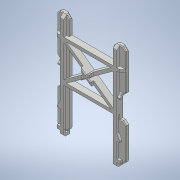
# Autodesk Inventor part: Крепление лидара
Saved by Autodesk Inventor 2020 (Build 240168000, 168)
## iProperties
Created: 2021-05-27
Part Number: Крепление лидара
Material: Типовые
Document SubType Name: Modeling
Designer: I_Love_U_Bogdan
Density: 1 g/cm^3
Appearance: По умолчанию
Author: I_Love_U_Bogdan
Autodesk Inventor part; units mm, degrees
ref_plane "YZ Plane" through (0, 0, 0) normal (1, 0, 0) x (0, 1, 0)
ref_plane "XZ Plane" through (0, 0, 0) normal (0, 1, 0) x (-1, 0, 0)
ref_plane "XY Plane" through (0, 0, 0) normal (0, 0, 1) x (1, 0, 0)
sketch "Эскиз1" plane through (0, 0, 0) normal (0, 0, 1) x (1, 0, 0)
  line L0 (-15, 85.8768) -> (-23, 85.8768)
  line L1 (-23, 85.8768) -> (-23, 17.8768)
  line L2 (-23, 17.8768) -> (-15, 17.8768)
  line L3 (-23.1, 75.8182) -> (-23.1, 81.8182) projected
  line L4 (-15, 85.8768) -> (-15, 17.8768)
  line L5 (-24.4209, 83.8768) -> (-19.4401, 83.8768) projected
  line L6 (-19.4401, 73.7596) -> (-24.4209, 73.7596) projected
  line L7 (-19.1, 75.8182) -> (-19.1, 81.8182) projected
  line L8 (-23, 57.8768) -> (-19, 57.8768)
  line L9 (-19, 57.8768) -> (-19, 42.8768)
  line L10 (-19, 42.8768) -> (-23, 42.8768)
  line L11 (-23, 42.8768) -> (-23, 57.8768)
  point P0 (0, 0)
  dimension "d0" = 0.1
  dimension "d1" = 68
  dimension "d2" = 8
  dimension "d3" = 2
  dimension "d4" = 10.1172
  dimension "d5" = 3.9
  dimension "d6" = 15
  dimension "d7" = 25
  constraints: 16 end point, 3 parallel, 2 horizontal, 2 perpendicular, 1 point on line
  measures "d0" distance between parallel lines of L3 L1
  measures "d1" distance of L0.end L1.end
  measures "d2" distance between parallel lines of L4 L1
  measures "d3" distance between parallel lines of L0 L5
  measures "d4" distance between parallel lines of L6 L5
  measures "d5" distance between parallel lines of L1 L7
  measures "d6" distance of L8.end L9.end
  measures "d7" distance between parallel lines of L2 L10
extrude "Выдавливание1" add sketch "Эскиз1" along normal blind 2 contours L4 L2 L1 L10 L9 L8 L0
sketch "Эскиз2" plane through (0, 0, 2) normal (0, 0, 1) x (1, 0, 0)
  line L0 (-19.4401, 73.7596) -> (-24.4209, 73.7596) projected
  line L1 (-23, 85.8768) -> (-23, 57.8768) projected
  line L2 (-23, 73.7596) -> (0, 73.7596)
  line L3 (0, 73.7596) -> (0, 71.7596)
  line L4 (0, 71.7596) -> (-23, 71.7596)
  line L5 (-23, 71.7596) -> (-23, 73.7596)
  line L6 (-15, 85.8768) -> (-23, 85.8768) projected
  line L7 (-15, 85.8768) -> (-16.5, 85.8768)
  line L8 (-16.5, 17.8768) -> (-15, 17.8768)
  line L9 (-19.1, 75.8182) -> (-19.1, 81.8182) projected
  line L10 (-25.5, 75.3182) -> (-26.5, 75.3182) projected
  line L11 (-23, 42.8768) -> (-23, 17.8768) projected
  line L12 (-23, 20.7596) -> (-19.1, 20.7596)
  line L13 (-25.5, 22.3182) -> (-26.5, 22.3182) projected
  line L14 (-26.5, 29.3182) -> (-25.5, 29.3182) projected
  line L15 (-23, 30.8768) -> (-19.1, 30.8768)
  line L16 (-16.5, 20.7596) -> (-21.1, 20.7596)
  line L17 (-21.1, 20.7596) -> (-21.1, 18.7596)
  line L18 (-21.1, 18.7596) -> (-16.5, 18.7596)
  line L19 (-23, 17.8768) -> (-15, 17.8768) projected
  line L20 (-16.5, 85.8768) -> (-19, 85.8768)
  line L21 (-19, 85.8768) -> (-19, 17.8768)
  line L22 (-19, 17.8768) -> (-16.5, 17.8768)
  line L23 (-16.5, 17.8768) -> (-16.5, 85.8768)
  line L24 (-21, 31.1768) -> (-21, 32.1768)
  line L25 (-21, 32.1768) -> (-19, 35.6409)
  line L26 (-16.5, 47.8768) -> (0, 47.8768)
  line L27 (0, 47.8768) -> (0, 45.8768)
  line L28 (0, 45.8768) -> (-16.5, 45.8768)
  line L29 (-16.5, 45.8768) -> (-16.5, 47.8768)
  line L30 (0, 71.7596) -> (0, 47.8768)
  line L31 (0, 59.8182) -> (-16.5, 47.8768) construction
  line L32 (-15.9137, 47.0667) -> (0.5863, 59.0081)
  arc A0 (0.5863, 59.0081) -> (0, 60.8182) centre (0, 59.8182) ccw
  arc A1 (-17.0863, 48.6869) -> (-15.9137, 47.0667) centre (-16.5, 47.8768) ccw
  line L33 (0, 59.8182) -> (-16.5, 71.7596) construction
  line L34 (0.5863, 60.6283) -> (-15.9137, 72.5697)
  arc A2 (0, 58.8182) -> (0.5863, 60.6283) centre (0, 59.8182) ccw
  arc A3 (-15.9137, 72.5697) -> (-17.0863, 70.9495) centre (-16.5, 71.7596) ccw
  line L35 (-17.0863, 70.9495) -> (-1.7056, 59.8182)
  line L36 (-1.7056, 59.8182) -> (-17.0863, 48.6869)
  line L37 (-21, 31.1768) -> (-19, 31.1768)
  line L38 (-19.1, 81.8182) -> (-19.1, 35.4676)
  line L39 (-19.1, 30.8768) -> (-19.1, 19.0812)
  point P0 (0, 0)
  point P1 (-8.25, 53.8475)
  point P2 (-8.25, 65.7889)
  point P3 (-16.5, 70.5252)
  point P4 (-16.5, 49.1112)
  point P5 (-14.7944, 71.7596)
  point P6 (-16.5, 73.7596)
  point P7 (-19, 20.7596)
  point P8 (-19, 18.7596)
  point P9 (-14.7944, 47.8768)
  point P10 (0, 58.5838)
  point P11 (0, 61.0526)
  point P12 (-19, 71.7596)
  point P13 (-19, 73.7596)
  dimension "d10" = 2
  dimension "d12" = 1.5586
  dimension "d13" = 1.5586
  dimension "d14" = 1.5586
  dimension "d15" = 2
  dimension "d16" = 0
  dimension "d18" = 2.5
  dimension "d22" = 30
  dimension "d23" = 1
  dimension "d24" = 2
  dimension "d25" = 2
  dimension "d26" = 2
  dimension "d27" = 28
  dimension "d30" = 0.3
  dimension "d56" = 0.1
  dimension "d57" = 0
  dimension "d59" = 2
  constraints: 66 end point, 16 point on line, 12 parallel, 9 perpendicular, 8 point on circle, 8 tangent, 5 horizontal, 4 centre point, 4 midpoint, 3 vertical
  measures "d10" distance of L2.end L3.end
  measures "d12" distance between parallel lines of L10 L0
  measures "d13" distance between parallel lines of L13 L12
  measures "d14" distance between parallel lines of L15 L14
  measures "d15" distance of L16.end L17.end
  measures "d16" distance between parallel lines of L12 L16
  measures "d18" distance between parallel lines of L23 L21
  measures "d22" angle of L25 L21
  measures "d23" distance of L24.start L24.end
  measures "d24" distance of L26.end L27.end
  measures "d25" diameter of A1
  measures "d26" diameter of A3
  measures "d27" distance between parallel lines of L19 L28
  measures "d30" distance between parallel lines of L15 L37
  measures "d56" distance between parallel lines of L21 L38
  measures "d57" horizontal distance of point (0, 0) L2.end
  measures "d59" distance between parallel lines of L21 L24
extrude "Выдавливание2" add sketch "Эскиз2" along normal blind 2 contours L2 L38 L4 L1 L0 | L2 L21 L4 L38 | L21 L6 L23 L2 | L2 L23 A3 L4 L21 | L2 L3 L4 L34 A3 L23 | L4 A3 L35 L23 L36 A1 L16 L21 | L25 L21 L37 L24 | A3 L34 L4 L23 | L23 L4 A3 | L4 L23 L35 A3 | L4 L34 L30 L32 L26 L23 L36 L35 | L21 L18 L17 L12 L16 | L16 L23 L18 L21 | L23 A1 L36 | L18 L23 L19 L21 | L26 L32 A1 L23 | L23 A1 L32 L26 L27 L28
sketch "Эскиз3" plane through (0, 0, 2) normal (0, 0, -1) x (-1, 0, 0)
  line L0 (16.5, 73.7596) -> (16.5, 85.8768) projected
  line L1 (16.5, 85.8768) -> (19, 85.8768) projected
  line L2 (19, 85.8768) -> (19, 73.7596) projected
  line L3 (19, 35.6409) -> (21, 32.1768) projected
  line L4 (21, 32.1768) -> (21, 31.1768) projected
  line L5 (21, 31.1768) -> (19, 31.1768) projected
  line L6 (19, 31.1768) -> (19, 20.7596) projected
  line L7 (19, 20.7596) -> (21.1, 20.7596) projected
  line L8 (21.1, 20.7596) -> (21.1, 18.7596) projected
  line L9 (21.1, 18.7596) -> (19, 18.7596) projected
  line L10 (19, 18.7596) -> (19, 17.8768) projected
  line L11 (19, 17.8768) -> (16.5, 17.8768) projected
  line L12 (16.5, 17.8768) -> (16.5, 45.8768) projected
  line L13 (16.5, 45.8768) -> (0, 45.8768) projected
  line L14 (0, 45.8768) -> (0, 47.8768) projected
  line L15 (0, 47.8768) -> (14.7944, 47.8768) projected
  line L16 (14.7944, 47.8768) -> (0, 58.5838) projected
  line L17 (0, 58.5838) -> (0, 61.0526) projected
  line L18 (0, 61.0526) -> (14.7944, 71.7596) projected
  line L19 (14.7944, 71.7596) -> (0, 71.7596) projected
  line L20 (0, 71.7596) -> (0, 73.7596) projected
  line L21 (0, 73.7596) -> (16.5, 73.7596) projected
  line L22 (1.7056, 59.8182) -> (16.5, 49.1112) projected
  line L23 (16.5, 49.1112) -> (16.5, 70.5252) projected
  line L24 (16.5, 70.5252) -> (1.7056, 59.8182) projected
  line L25 (15, 73.7596) -> (15, 85.8768) projected
  line L26 (15, 50.1967) -> (15, 69.4396) projected
  line L27 (15, 17.8768) -> (15, 45.8768) projected
  line L28 (15, 69.4396) -> (15, 73.7596) projected
  line L29 (15, 73.7596) -> (15, 45.8768)
  line L30 (15, 17.8768) -> (15, 85.8768) projected
  line L31 (19, 73.7596) -> (23, 73.7596) projected
  line L32 (23, 73.7596) -> (23, 71.7596) projected
  line L33 (23, 71.7596) -> (19, 71.7596) projected
  line L34 (19, 71.7596) -> (19, 35.6409) projected
  point P0 (0, 0)
  point P1 (15, 71.7596)
  point P2 (14.8, 47.8768)
  point P3 (14.8, 48.3873)
  point P4 (15, 50.1967)
  point P5 (14.8, 71.2491)
  constraints: 2 end point, 1 collinear
extrude "Выдавливание3" add sketch "Эскиз3" along normal blind 2 contours L0 L1 L2 L31 L32 L33 L34 L3 L4 L5 L6 L7 L8 L9 L10 L11 L12 L13 L29 L22 L23 L24 L28 L21 | L28 L24 L22 L29 L13 L14 L15 L16 L17 L18 L19 L20 L21 | L24 L23 L22 L26
chamfer "Фаска1" distance 2 angle 45 8 edges at (-23, 72.7596, 4) (-23, 85.8768, 1) (-17.75, 85.8768, 4) (-15, 85.8768, 1) (-15, 17.8768, 1) (-23, 17.8768, 1) (-23, 57.8768, 1) (-23, 42.8768, 1)
chamfer "Фаска2" distance 0.5 angle 45 17 edges at (-23, 78.8182, 2) (-23, 65.8182, 2) (-23, 30.3768, 2) (-22, 84.8768, 2) (-20, 85.8768, 2) (-15.75, 84.6268, 2) (-22, 84.8768, 0) (-16, 84.8768, 0) (-22, 18.8768, 0) (-22, 18.8768, 2) (-20, 17.8768, 2) (-15.75, 19.1268, 2) (-16, 18.8768, 0) (-20, 42.8768, 2) (-22, 41.8768, 2) (-20, 57.8768, 2) (-22, 58.8768, 2)
sketch "Эскиз7" plane through (-19, 17.8768, 4) normal (0, -1, 0) x (1, 0, 0)
  line L0 (2, -3.5) -> (1.2929, -4) projected
  line L1 (2, 0) -> (2, -3.5) projected
  line L2 (0, 0) -> (2, 0) projected
  line L3 (0, -2.5) -> (0, 0) projected
  line L4 (-2, -2.5) -> (0, -2.5) projected
  line L5 (-2, -3.5) -> (-2, -2.5) projected
  line L6 (-1.2929, -4) -> (-2, -3.5) projected
  line L7 (-1.2929, -4) -> (1.2929, -4) projected
  line L8 (0, 0) -> (2.5, 0) projected
  line L9 (4, -4) -> (1.2929, -4) projected
  line L10 (0, 0) -> (2.5231, 0)
  line L11 (2.5231, 0) -> (2.5231, -4)
  line L12 (2.5231, -4) -> (0, -4)
  line L13 (0, -4) -> (0, 0)
  point P0 (19, -4)
  point P1 (0, -4)
  constraints: 8 end point, 2 parallel, 1 horizontal, 1 perpendicular, 1 point on line
extrude "Выдавливание7" add sketch "Эскиз7" along normal mid plane 4 contours L1 L8 L10 L11 L9 L0 | L0 L7 L13 L3 L2 L1
chamfer "Фаска3" distance 1 angle 45 1 edges at (-17.7385, 15.8768, 4)
sketch "Эскиз4" plane through (-19, 20.7596, 2) normal (-1, 0, 0) x (0, 0, 1)
  line L0 (-2, 25.1172) -> (2, 25.1172) projected
  line L1 (-0.5, -2.8828) -> (2, -2.8828) projected
  line L2 (0, 25.1172) -> (0.6, 25.1172)
  line L3 (0.6, 25.1172) -> (0.6, -2.8828)
  line L4 (0.6, -2.8828) -> (0, -2.8828)
  line L5 (0, -2.8828) -> (0, 25.1172)
  line L6 (0, -2.3828) -> (-0.5, -2.8828) projected
  line L7 (-1.5, -2.8828) -> (-0.5, -2.8828) projected
  line L8 (-1.5, -3.2828) -> (-0.5, -3.2828)
  line L9 (0, -2.8828) -> (0, -3.2828)
  line L10 (0, -3.2828) -> (-0.5, -3.2828)
  line L11 (0.6, -2.8828) -> (0.6, -3.2828)
  line L12 (0.6, -3.2828) -> (0, -3.2828)
  line L13 (-1.5, -3.2828) -> (-2, -3.2828)
  line L14 (-2, -2.8828) -> (-2, -4.8828) projected
  line L15 (2, 63.1172) -> (2, 53) projected
  line L16 (0, -2) -> (2, -2) projected
  line L17 (0, -2.3828) -> (0, -2) projected
  line L18 (-2, -2.8828) -> (-0.5, -2.8828) projected
  line L19 (2, -3.8828) -> (1, -4.8828) projected
  line L20 (2, -2) -> (2, -3.8828) projected
  line L21 (-0.5, -2.8828) -> (0, -2.3828) projected
  line L22 (-2, -2.8828) -> (-2, -4.8828) projected
  line L23 (1, -4.8828) -> (-2, -4.8828) projected
  line L24 (0, 0) -> (0, 10.4172) projected
  line L25 (0, 0) -> (2, 0) projected
  line L26 (2, 10.4172) -> (2, 0) projected
  line L27 (0, 10.4172) -> (2, 10.4172) projected
  line L28 (0, 65.1172) -> (2, 63.1172) projected
  line L29 (0, 65.1172) -> (-0.5, 65.1172) projected
  line L30 (-0.5, 65.1172) -> (0, 64.6172) projected
  line L31 (0, 53) -> (0, 64.6172) projected
  line L32 (0, 53) -> (2, 53) projected
  line L33 (0, 14.8813) -> (0, 21.6172) projected
  line L34 (0, 14.8813) -> (2, 14.8813) projected
  line L35 (2, 51) -> (2, 14.8813) projected
  line L36 (0, 51) -> (2, 51) projected
  line L37 (0, 37.6172) -> (0, 51) projected
  line L38 (-0.5, 37.1172) -> (0, 37.6172) projected
  line L39 (-2, 37.1172) -> (-0.5, 37.1172) projected
  line L40 (-2, 37.1172) -> (-2, 22.1172) projected
  line L41 (-2, 22.1172) -> (-0.5, 22.1172) projected
  line L42 (0, 21.6172) -> (-0.5, 22.1172) projected
  point P0 (-2, -20.7596)
  point P1 (0, -2.8828)
  point P2 (-1.5, -2.8828)
  point P3 (-2, -2.8828)
  dimension "d39" = 0.6
  dimension "d48" = 0.4
  constraints: 20 end point, 4 perpendicular, 4 point on line, 3 parallel, 1 horizontal, 1 midpoint, 1 vertical
  measures "d39" distance of L3.end L4.end
  measures "d48" distance between parallel lines of L7 L8
extrude "Выдавливание4" cut sketch "Эскиз4" against normal through all both and the other way through all contours L0 L3 L34 L5 | L3 L27 L5 L34 | L3 L25 L5 L27 | L3 L16 L5 L25 | L3 L1 L5 L16 | L11 L12 L9 L1 | L5 L1 L6 | L9 L10 L8 L13 L14 L18 L7 L1
chamfer "Фаска4" distance 0.5 angle 45 1 edges at (-17.7385, 17.4768, 2.6)
sketch "Эскиз8" plane through (-21, 57.8768, 1.5) normal (0, -0.7071068, 0.7071068) x (1, 0, 0)
  line L0 (0, 0) -> (2, 0) projected
  line L1 (2, 0) -> (2, 0.7071) projected
  line L2 (2, 0.7071) -> (0.2071, 0.7071) projected
  line L3 (0.2071, 0.7071) -> (0, 0) projected
  point P0 (21, -41.9857)
extrude "Выдавливание8" add sketch "Эскиз8" along normal blind 3
chamfer "Фаска5" distance 0.5 angle 45 1 edges at (-19.8964, 56.2554, 4.1213)
chamfer "Фаска6" distance 1 angle 45 1 edges at (-19.8964, 58.3768, 2)
mirror "Зеркальное отражение1" about plane through (0, 58.5838, 2) normal (1, 0, 0)
sketch "Эскиз6" plane through (0, 0, 4) normal (0, 0, 1) x (1, 0, 0)
  line L0 (14.7944, 47.8768) -> (0, 58.5838) projected
  line L1 (0, 61.0526) -> (-14.7944, 71.7596) projected
  line L2 (0, 58.5838) -> (0, 61.0526)
  line L3 (3.5, 63.8182) -> (-3.5, 63.8182)
  line L4 (-3.5, 63.8182) -> (-3.5, 55.8182)
  line L5 (-3.5, 55.8182) -> (3.5, 55.8182)
  line L6 (3.5, 55.8182) -> (3.5, 63.8182)
  line L7 (3.5, 63.8182) -> (-3.5, 55.8182) construction
  line L8 (-3.5, 63.8182) -> (3.5, 55.8182) construction
  line L9 (-14.7944, 47.8768) -> (14.7944, 47.8768) projected
  line L10 (-14.7944, 47.8768) -> (0, 58.5838) projected
  line L11 (14.7944, 47.8768) -> (0, 58.5838) projected
  line L12 (-16.5, 45.8768) -> (16.5, 45.8768) projected
  line L13 (16.5, 19.8768) -> (16.5, 45.8768) projected
  line L14 (19, 18.7596) -> (19, 16.8768) projected
  line L15 (21.1, 18.7596) -> (19, 18.7596) projected
  line L16 (21.1, 20.7596) -> (21.1, 18.7596) projected
  line L17 (19, 20.7596) -> (21.1, 20.7596) projected
  line L18 (19, 31.1768) -> (19, 20.7596) projected
  line L19 (21, 31.1768) -> (19, 31.1768) projected
  line L20 (21, 32.1768) -> (21, 31.1768) projected
  line L21 (19, 35.6409) -> (21, 32.1768) projected
  line L22 (21, 71.7596) -> (19, 71.7596) projected
  line L23 (21, 71.7596) -> (21, 73.7596) projected
  line L24 (19, 73.7596) -> (21, 73.7596) projected
  line L25 (19, 83.8768) -> (19, 73.7596) projected
  line L26 (19, 83.8768) -> (16.5, 83.8768) projected
  line L27 (16.5, 73.7596) -> (16.5, 83.8768) projected
  line L28 (-16.5, 73.7596) -> (16.5, 73.7596) projected
  line L29 (-16.5, 73.7596) -> (-16.5, 83.8768) projected
  line L30 (-19, 83.8768) -> (-16.5, 83.8768) projected
  line L31 (-19, 83.8768) -> (-19, 73.7596) projected
  line L32 (-19, 73.7596) -> (-21, 73.7596) projected
  line L33 (-21, 71.7596) -> (-21, 73.7596) projected
  line L34 (-21, 71.7596) -> (-19, 71.7596) projected
  line L35 (-19, 35.6409) -> (-21, 32.1768) projected
  line L36 (-21, 32.1768) -> (-21, 31.1768) projected
  line L37 (-21, 31.1768) -> (-19, 31.1768) projected
  line L38 (-19, 31.1768) -> (-19, 20.7596) projected
  line L39 (-19, 20.7596) -> (-21.1, 20.7596) projected
  line L40 (-21.1, 20.7596) -> (-21.1, 18.7596) projected
  line L41 (-21.1, 18.7596) -> (-19, 18.7596) projected
  line L42 (-19, 71.7596) -> (-19, 35.6409) projected
  line L43 (-16.5, 19.8768) -> (-16.5, 45.8768) projected
  line L44 (16.5, 49.1112) -> (16.5, 70.5252) projected
  line L45 (1.7056, 59.8182) -> (16.5, 49.1112) projected
  line L46 (16.5, 70.5252) -> (1.7056, 59.8182) projected
  line L47 (-14.7944, 71.7596) -> (14.7944, 71.7596) projected
  line L48 (0, 61.0526) -> (14.7944, 71.7596) projected
  line L49 (0, 61.0526) -> (-14.7944, 71.7596) projected
  line L50 (-16.5, 49.1112) -> (-16.5, 70.5252) projected
  line L51 (-16.5, 70.5252) -> (-1.7056, 59.8182) projected
  line L52 (-1.7056, 59.8182) -> (-16.5, 49.1112) projected
  line L53 (16.5, 19.8768) -> (16.4769, 19.8768) projected
  line L54 (16.4769, 16.8768) -> (16.4769, 19.8768) projected
  line L55 (16.4769, 16.8768) -> (19, 16.8768) projected
  line L56 (-16.4769, 16.8768) -> (-19, 16.8768) projected
  line L57 (-16.4769, 16.8768) -> (-16.4769, 19.8768) projected
  line L58 (-16.5, 19.8768) -> (-16.4769, 19.8768) projected
  line L59 (19, 71.7596) -> (19, 35.6409) projected
  line L60 (-19, 18.7596) -> (-19, 16.8768) projected
  point P0 (0, 0)
  point P1 (0, 59.8182)
  point P2 (3.5, 56.0507)
  point P3 (3.5, 58.6174)
  point P4 (3.5, 61.019)
  point P5 (3.5, 63.4492)
  point P6 (-3.5, 63.5856)
  point P7 (-3.5, 61.019)
  point P8 (-3.5, 58.6174)
  point P9 (-3.5, 56.1872)
  point P10 (-3.5, 63.5856)
  point P11 (3.5, 63.5856)
  point P12 (3.5, 56.0507)
  point P13 (-3.5, 56.0507)
  point P14 (3.5, 61.1168)
  point P15 (3.5, 58.5196)
  point P16 (-3.5, 58.5196)
  point P17 (-3.5, 61.1168)
  dimension "d52" = 7
  dimension "d53" = 8
  constraints: 14 end point, 3 midpoint, 2 parallel, 1 horizontal, 1 perpendicular, 1 vertical
  measures "d52" distance of L5.end L4.end
  measures "d53" distance of L4.end L3.end
extrude "Выдавливание6" add sketch "Эскиз6" along normal blind 2 contours L0 L2 L48 L6 L46 L45 | L10 L4 L52 L51 L1 L2
chamfer "Фаска7" distance 0.5 angle 45 12 edges at (-3.5, 62.3512, 6) (-3.5, 57.2851, 6) (3.5, 62.3512, 6) (3.5, 57.2851, 6) (-2.6028, 60.4675, 6) (-2.6028, 59.1689, 6) (2.6028, 60.4675, 6) (2.6028, 59.1689, 6) (1.75, 57.3172, 6) (-1.75, 57.3172, 6) (-1.75, 62.3191, 6) (1.75, 62.3191, 6)
equation "\"d13\" = d12"
equation "\"d14\" = d13"
